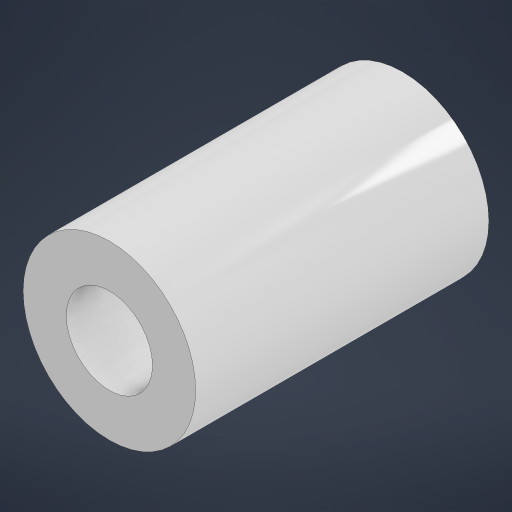
# Autodesk Inventor part: multif_lvl_spacer
Saved by Autodesk Inventor 2024 (Build 280153000, 153)
## iProperties
Created: 2026-03-28
Part Number: multif_lvl_spacer
Material: PET Plastic
Document SubType Name: Modeling
Designer: schar
Density: 1.541 g/cm^3
Appearance: Polycarbonate - Clear
Author: schar
Autodesk Inventor part; units mm, degrees
ref_plane "YZ Plane" through (0, 0, 0) normal (1, 0, 0) x (0, 1, 0)
ref_plane "XZ Plane" through (0, 0, 0) normal (0, 1, 0) x (-1, 0, 0)
ref_plane "XY Plane" through (0, 0, 0) normal (0, 0, 1) x (1, 0, 0)
sketch "Sketch1" plane through (0, 0, 0) normal (0, 0, 1) x (1, 0, 0)
  circle A0 centre (-72.399, 16.2222) radius 1.5 projected
  circle A1 centre (-71.8393, -17.5564) radius 1.5 projected
  line L0 (-78.8983, 31.2807) -> (-56.1772, 18.6414) projected
  line L1 (-56.1772, 18.6414) -> (-65.2012, 2.4193) projected
  line L2 (-65.2012, 2.4193) -> (-65.2248, -2.3776) projected
  line L3 (-65.2248, -2.3776) -> (-55.5023, -19.8554) projected
  line L4 (-55.5023, -19.8554) -> (-58.1004, -21.3554) projected
  line L5 (-58.1004, -21.3554) -> (-75.5782, -31.0779) projected
  line L6 (-75.5782, -31.0779) -> (-78.1762, -32.5779) projected
  line L7 (-78.1762, -32.5779) -> (-95.6183, -1.7293) projected
  line L8 (-95.6183, -1.7293) -> (-95.6284, 1.2056) projected
  line L9 (-95.6284, 1.2056) -> (-78.8983, 31.2807) projected
  circle A2 centre (-81.423, 0) radius 2.5 projected
  circle A3 centre (-81.4228, 0.0001) radius 5 projected
  point P0 (0, 0)
extrude "Extrusion1" add sketch "Sketch1" along normal blind 17 contours A3
body "Solid1"
